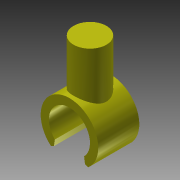
# Autodesk Inventor part: HAND
Saved by Autodesk Inventor 2015 (Build 190159000, 159)
## iProperties
Created: 2012-05-01
Part Number: HAND
Material: 250
Document SubType Name: Modeling
Mass: 0.140052 g
Surface Area: 0.635869 cm^2
Volume: 0.017841 cm^3
Density: 7.85 g/cm^3
Appearance: Steel
Autodesk Inventor part; units mm, degrees
ref_plane "YZ Plane" through (0, 0, 0) normal (1, 0, 0) x (0, 1, 0)
ref_plane "XY Plane" through (0, 0, 0) normal (0, 0, 1) x (1, 0, 0)
sketch "Sketch1" plane through (0, 0, 0) normal (0, 0, 1) x (1, 0, 0)
  circle A0 centre (0, 0) radius 1.75
  circle A1 centre (0, 0) radius 1.25
  line L0 (-0.89, -0.8777) -> (-0.975, -1.4532)
  line L1 (0.89, -0.8777) -> (0.975, -1.4532)
  dimension "d0" = 3.5
  dimension "d1" = 2.5
  dimension "d2" = 1.95
  dimension "d3" = 1.78
  constraints: 4 end point, 4 point on circle, 2 centre point, 2 coincident, 2 horizontal alignment
  measures "d0" diameter of A0
  measures "d1" diameter of A1
  measures "d2" distance of L1.end L0.end
  measures "d3" distance of L1.start L0.start
extrude "Extrusion1" add sketch "Sketch1" along normal mid plane 2.5 contours A0 L1 A1 L0 picked at (1.5663, 0.14)
chamfer "Chamfer1" distance 0.2 angle 45 2 edges at (-0.975, -1.4532, 0) (0.975, -1.4532, 0)
ref_plane "Work Plane1" through (0, 4.436, 0) normal (0, 1, 0) x (-1, 0, 0)
sketch "Sketch2" plane through (0, 4.436, 0) normal (0, 1, 0) x (-1, 0, 0)
  circle A0 centre (0, 0) radius 1
  dimension "d10" = 2
  constraints: 1 centre point, 1 coincident
  measures "d10" diameter of A0
extrude "Extrusion2" add sketch "Sketch2" against normal up to surface
body "Solid1"
